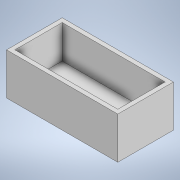
# Autodesk Inventor part: obudowa_latarka_gora
Saved by Autodesk Inventor 2020.4 (Build 244396000, 396)
## iProperties
Created: 2021-06-08
Part Number: obudowa_latarka_gora
Material: Ogólny
Document SubType Name: Modeling
Designer: przem
Density: 1 g/cm^3
Appearance: Domyślna
Author: przem
Autodesk Inventor part; units mm, degrees
ref_plane "YZ Plane" through (0, 0, 0) normal (1, 0, 0) x (0, 1, 0)
ref_plane "XZ Plane" through (0, 0, 0) normal (0, 1, 0) x (-1, 0, 0)
ref_plane "XY Plane" through (0, 0, 0) normal (0, 0, 1) x (1, 0, 0)
sketch "Szkic1" plane through (0, 0, 0) normal (0, 1, 0) x (-1, 0, 0)
  line L0 (0, 0) -> (40, 0)
  line L1 (40, 0) -> (40, -20)
  line L2 (40, -20) -> (0, -20)
  line L3 (0, -20) -> (0, 0)
  dimension "d0" = 40
  dimension "d1" = 20
  constraints: 8 end point, 2 parallel, 1 horizontal, 1 perpendicular
  measures "d0" distance of L1.end L2.end
  measures "d1" distance of L0.end L1.end
extrude "Wyciągnięcie proste1" add sketch "Szkic1" along normal blind 15
sketch "Szkic2" plane through (0, 15, 0) normal (0, 1, 0) x (1, 0, 0)
  line L0 (-40, 0) -> (0, 0) construction
  line L1 (0, 0) -> (0, 1.5) construction
  line L2 (0, 0) -> (0, 20) construction
  line L3 (0, 1.5) -> (-1.5, 1.5) construction
  line L4 (-1.5, 1.5) -> (-38.5, 1.5)
  line L5 (-38.5, 1.5) -> (-38.5, 18.5)
  line L6 (-38.5, 18.5) -> (-1.5, 18.5)
  line L7 (-1.5, 18.5) -> (-1.5, 1.5)
  dimension "d4" = 1.5
  dimension "d5" = 1.5
  dimension "d6" = 37
  dimension "d7" = 17
  constraints: 12 end point, 2 parallel, 2 perpendicular, 1 horizontal, 1 point on line
  measures "d4" distance of L0.end L1.end
  measures "d5" distance of L1.end L3.end
  measures "d6" distance of L5.end L6.end
  measures "d7" distance of L4.end L5.end
extrude "Wyciągnięcie proste2" cut sketch "Szkic2" against normal blind 12
sketch "Szkic3" plane through (-40, 0, 0) normal (0, 0, 1) x (1, 0, 0)
  line L0 (1.5, 3) -> (38.5, 3) projected
  line L1 (38.5, 15) -> (38.5, 3) projected
  line L2 (1.5, 3) -> (38.5, 3)
  line L3 (38.5, 3) -> (38.5, 15)
  line L4 (1.5, 15) -> (1.5, 3)
  line L5 (1.5, 15) -> (1.5, 3) construction
  line L6 (38.5, 15) -> (20, 15)
  line L7 (0, 15) -> (40, 15) projected
  line L8 (20, 15) -> (20, 10)
  line L9 (18, 9.5) -> (22, 9.5)
  line L10 (22, 9.5) -> (22, 10.5)
  line L11 (22, 10.5) -> (18, 10.5)
  line L12 (18, 10.5) -> (18, 9.5)
  line L13 (18, 9.5) -> (22, 10.5) construction
  line L14 (22, 9.5) -> (18, 10.5) construction
  point P0 (40, 0)
  dimension "d13" = 5
  dimension "d14" = 4
  dimension "d15" = 1
  constraints: 22 end point, 3 midpoint, 3 parallel, 3 perpendicular, 2 horizontal
  measures "d13" distance of L6.end L8.end
  measures "d14" distance of L11.end L10.end
  measures "d15" distance of L10.end L9.end
extrude "Wyciągnięcie proste3" add sketch "Szkic3" against normal blind 2.3 contours L11 L10 L9 L12
equation "\"d6\" = d0 - 2 * d5"
equation "\"d7\" = d1 - 2 * d5"
